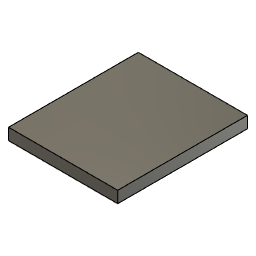
lid_lid v1 (Autodesk Fusion 360 design; units mm, degrees)
Autodesk Fusion 360 part; units mm, degrees
sketch "Sketch1" plane through (0, 0, 0) normal (0, 1, 0) x (1, 0, 0)
  line L0 (-35.75, 41.5) -> (-33.75, 41.5)
  line L1 (-33.75, 41.5) -> (-33.75, -41.5)
  line L2 (-33.75, -41.5) -> (33.75, -41.5)
  line L3 (33.75, -41.5) -> (33.75, 41.5)
  line L4 (33.75, 41.5) -> (35.75, 41.5)
  line L5 (35.75, 41.5) -> (35.75, -43.5)
  line L6 (35.75, -43.5) -> (-35.75, -43.5)
  line L7 (-35.75, -43.5) -> (-35.75, 41.5)
  dimension "d1" = 2
  dimension "d2" = 2
  dimension "d3" = 2
  dimension "d4" = 67.5
  dimension "d5" = 83
  dimension "d6" = 33.75
  dimension "d7" = 41.5
  constraint horizontal L0
  constraint perpendicular L0 L1
  constraint perpendicular L1 L2
  constraint perpendicular L2 L3
  constraint perpendicular L3 L4
  constraint perpendicular L2 L5
  constraint perpendicular L5 L6
  constraint parallel L1 L7
  constraint collinear L0 L4
  measures "d1" distance of L1 L7
  measures "d2" distance of L3 L5
  measures "d3" distance of L2 L6
  measures "d4" distance of L1 L3
  measures "d5" distance of L0.end L1.end
  measures "d6" distance of origin L3
  measures "d7" distance of origin L2
extrude "Extrude1" add sketch "Sketch1" along normal blind 5.1
sketch "Sketch2" plane through (0, 5.1, 0) normal (0, 1, 0) x (-1, 0, 0)
  line L0 (35.75, 43.5) -> (-35.75, 43.5)
  line L1 (-35.75, 43.5) -> (-35.75, -41.5)
  line L2 (-35.75, -41.5) -> (-33.75, -41.5)
  line L3 (-33.75, -41.5) -> (-33.75, 41.5)
  line L4 (-33.75, 41.5) -> (33.75, 41.5)
  line L5 (33.75, 41.5) -> (33.75, -41.5)
  line L6 (33.75, -41.5) -> (35.75, -41.5)
  line L7 (35.75, -41.5) -> (35.75, 43.5)
  line L8 (35.75, 43.5) -> (-35.75, 43.5)
  line L9 (-35.75, 43.5) -> (-35.75, -41.5)
  line L10 (-35.75, -41.5) -> (35.75, -41.5)
  line L11 (35.75, -41.5) -> (35.75, 43.5)
  constraint horizontal L8
  constraint vertical L9
  constraint horizontal L10
  constraint vertical L11
  constraint coincident L1.end L2.start
  constraint coincident L0.start L7.end
extrude "Extrude2" add sketch "Sketch2" along normal blind 2.5
equation "d2 = d1"
equation "d3 = d1"
equation "d4 = 60 mm + 6 mm + 1.5 mm"
equation "d5 = 80 mm + 3 mm"
equation "d6 = d4 / 2"
equation "d7 = d5 / 2"
